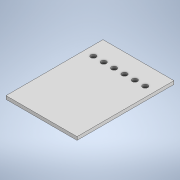
# Autodesk Inventor part: sheild
Saved by Autodesk Inventor 2021 (Build 250183000, 183)
## iProperties
Created: 2021-01-28
Part Number: sheild
Material: Generic
Document SubType Name: Modeling
Designer: Ryan
Density: 1 g/cm^3
Appearance: Default
Author: Ryan
Autodesk Inventor part; units mm, degrees
ref_plane "YZ Plane" through (0, 0, 0) normal (1, 0, 0) x (0, 1, 0)
ref_plane "XZ Plane" through (0, 0, 0) normal (0, 1, 0) x (-1, 0, 0)
ref_plane "XY Plane" through (0, 0, 0) normal (0, 0, 1) x (1, 0, 0)
sketch "Sketch1" plane through (0, 0, 0) normal (0, 1, 0) x (-1, 0, 0)
  line L0 (34.798, 47.498) -> (-34.798, 47.498)
  line L1 (-34.798, 47.498) -> (-34.798, -47.498)
  line L2 (-34.798, -47.498) -> (34.798, -47.498)
  line L3 (34.798, -47.498) -> (34.798, 47.498)
  point P0 (0, 0)
  dimension "d0" = 47.498
  dimension "d1" = 94.996
  dimension "d2" = 69.596
  dimension "d3" = 34.798
  constraints: 8 end point, 2 parallel, 1 horizontal, 1 perpendicular
  measures "d0" distance from line of point (0, 0) L2
  measures "d1" distance of L2.end L0.start
  measures "d2" distance of L1.end L2.end
  measures "d3" distance from line of L3 point (0, 0)
extrude "Extrusion1" add sketch "Sketch1" along normal blind 3.175
sketch "Sketch2" plane through (0, 3.175, 0) normal (0, 1, 0) x (1, 0, 0)
  line L0 (-34.798, -47.498) -> (34.798, -47.498) projected
  line L1 (0, -47.498) -> (0, 28.702) construction
  line L2 (-34.798, 47.498) -> (-34.798, -47.498) projected
  line L3 (-34.798, 28.702) -> (32.4262, 28.702) construction
  circle A0 centre (-5.08, 28.702) radius 2.54
  circle A1 centre (-15.24, 28.702) radius 2.54
  circle A2 centre (-25.4, 28.702) radius 2.54
  circle A3 centre (5.08, 28.702) radius 2.54
  circle A4 centre (15.24, 28.702) radius 2.54
  circle A5 centre (25.4, 28.702) radius 2.54
  point P0 (0, 0)
  dimension "d6" = 5.08
  dimension "d7" = 10.16
  dimension "d8" = 10.16
  dimension "d9" = 76.2
  dimension "d10" = 5.08
  constraints: 6 centre point, 5 point on line, 4 end point, 3 midpoint, 3 symmetric about line, 2 equal radius, 1 perpendicular, 1 vertical, 3 other
  measures "d6" distance from line of L1 A0.centre
  measures "d7" distance of A1.centre A0.centre
  measures "d8" distance of A2.centre A1.centre
  measures "d9" distance of L1.start L1.end
  measures "d10" diameter of A2
extrude "Extrusion2" cut sketch "Sketch2" against normal blind 3.175
equation "\"d0\" = 0.5 * d1"
equation "\"d3\" = 0.5 * d2"
body "Solid1"
